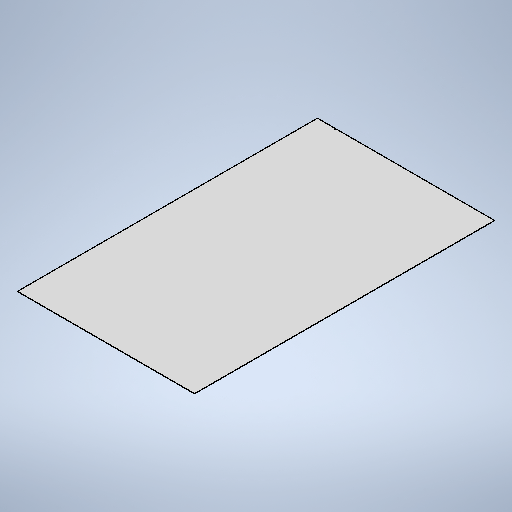
# Autodesk Inventor part: GnG frame 1.1 floor sheet 4
Saved by Autodesk Inventor 2025.3 (Build 293356000, 356)
## iProperties
Created: 2025-10-28
Part Number: GnG frame 1.1 floor sheet 4
Material: Stainless Steel
Document SubType Name: Sheet Metal
Designer: admin
Mass: 280.619 g
Surface Area: 364.406 cm^2
Volume: 35.0774 cm^3
Density: 8 g/cm^3
Sheet Metal Rule: AISI304 3mm Die 32
Sheet Metal Width: 1240,000 mm
Sheet Metal Length: 2100,000 mm
Sheet Metal Area: 2604000,000 mm^2
Appearance: Default
Stock Number: 1.4
Flat Pattern Width: 124 cm
Flat Pattern Length: 210 cm
Flat Pattern Area: 26040 cm^2
Author: admin
Autodesk Inventor part; units mm, degrees
ref_plane "YZ Plane" through (0, 0, 0) normal (1, 0, 0) x (0, 1, 0)
ref_plane "XZ Plane" through (0, 0, 0) normal (0, 1, 0) x (-1, 0, 0)
ref_plane "XY Plane" through (0, 0, 0) normal (0, 0, 1) x (1, 0, 0)
sketch "Sketch1" plane through (0, 0, 0) normal (0, 0, 1) x (1, 0, 0)
  line L0 (0, 0) -> (-1240, 0)
  line L1 (-1240, 0) -> (-1240, -2100)
  line L2 (-1240, -2100) -> (0, -2100)
  line L3 (0, -2100) -> (0, 0)
  line L4 (0, 0) -> (-35, 0)
  line L5 (-35, 0) -> (-35, -35)
  line L6 (-35, -35) -> (0, -35)
  line L7 (0, -35) -> (0, 0)
  line L8 (0, -2100) -> (-35, -2100)
  line L9 (-35, -2100) -> (-35, -2065)
  line L10 (-35, -2065) -> (0, -2065)
  line L11 (0, -2065) -> (0, -2100)
  line L12 (-1240, 0) -> (-1205, 0)
  line L13 (-1205, 0) -> (-1205, -35)
  line L14 (-1205, -35) -> (-1240, -35)
  line L15 (-1240, -35) -> (-1240, 0)
  line L16 (-1240, -2100) -> (-1205, -2100)
  line L17 (-1205, -2100) -> (-1205, -2065)
  line L18 (-1205, -2065) -> (-1240, -2065)
  line L19 (-1240, -2065) -> (-1240, -2100)
  line L20 (-1095, -2100) -> (-1005, -2100)
  line L21 (-1005, -2100) -> (-1005, -2065)
  line L22 (-1005, -2065) -> (-1095, -2065)
  line L23 (-1095, -2065) -> (-1095, -2100)
  line L24 (-1095, 0) -> (-1005, 0)
  line L25 (-1005, 0) -> (-1005, -35)
  line L26 (-1005, -35) -> (-1095, -35)
  line L27 (-1095, -35) -> (-1095, 0)
  point P0 (0, -35)
  point P1 (0, -2065)
  point P2 (-1005, -2100)
  point P3 (-1005, 0)
  dimension "d22" = 1240
  dimension "d23" = 2100
  dimension "d24" = 35
  dimension "d25" = 35
  dimension "d28" = 90
  dimension "d29" = 970
  measures "d22" distance of L2.end L1.end
  measures "d23" distance of L1.end L0.end
  measures "d24" distance of L6.end L5.end
  measures "d25" distance of L5.end L4.end
  measures "d28" distance of L25.end L26.end
  measures "d29" distance between parallel lines of L5 L25
extrude "Plate1" add sketch "Sketch1" along normal blind 3
sketch "Sketch5" plane through (0, 0, 3) normal (0, 0, 1) x (1, 0, 0)
  line L0 (-1135, 0) -> (-1133, 0)
  line L1 (-1131, 0) -> (-1129, 0)
  circle A0 centre (-1140, 0) radius 1.5
  line L2 (-1125, 0) -> (-1125, -5)
  line L3 (-1123, 0) -> (-1121.9884, -4.6072)
  arc A1 (-1121.9884, -4.6072) -> (-1121.0116, -4.6072) centre (-1121.5, -4.5) ccw
  line L4 (-1123, 0) -> (-1120, 0)
  line L5 (-1125, 0) -> (-1123, 0) construction
  line L6 (-1120, 0) -> (-1118, 0) construction
  line L7 (-1121.0116, -4.6072) -> (-1120, 0)
  line L8 (-1118, -5) -> (-1118, 0)
  line L9 (-1118, 0) -> (-1116, 0)
  line L10 (-1116, 0) -> (-1116, -5)
  line L11 (-1116, -5) -> (-1118, -5)
  line L12 (-1116, -2.5) -> (-1114, -2.5) construction
  line L13 (-1129, -5) -> (-1131, -5)
  line L14 (-1125, -5) -> (-1127, -5)
  line L15 (-1129, -2.5) -> (-1127, -2.5) construction
  line L16 (-1133, -2.5) -> (-1131, -2.5) construction
  line L17 (-1127, 0) -> (-1125, 0)
  line L18 (-1127, -5) -> (-1127, 0)
  line L19 (-1129, 0) -> (-1129, -5)
  line L20 (-1131, -5) -> (-1131, 0)
  line L21 (-1133, 0) -> (-1133, -5)
  line L22 (-1135, -5) -> (-1135, 0)
  line L23 (-1133, -5) -> (-1135, -5)
  line L24 (-1114, -5) -> (-1114, 0)
  line L25 (-1112, -5) -> (-1114, -5)
  line L26 (-1114, 0) -> (-1112, 0)
  line L27 (-1112, 0) -> (-1112, -5)
  line L28 (-1112, -2.5) -> (-1110, -2.5) construction
  line L29 (-1110, -5) -> (-1110, 0)
  line L30 (-1110, 0) -> (-1108, 0)
  line L31 (-1108, 0) -> (-1108, -5)
  line L32 (-1108, -5) -> (-1110, -5)
  line L33 (-1240, 0) -> (0, 0) projected
  line L34 (-1104, -5) -> (-1106, -5)
  line L35 (-1106, -5) -> (-1106, 0)
  line L36 (-1104, 0) -> (-1104, -5)
  line L37 (-1106, 0) -> (-1104, 0)
  line L38 (-1106, -2.5) -> (-1108, -2.5)
  point P0 (-1121.5, 0)
  point P1 (-1105, 0)
  point P2 (-1104, 0)
  point P3 (-1106, 0)
  dimension "d30" = 2
  dimension "d31" = 5
  dimension "d32" = 0.5
  dimension "d33" = 3
  dimension "d34" = 2
  dimension "d35" = 5
  dimension "d36" = 3
  dimension "d37" = 5
  dimension "d38" = 100
  constraints: 76 end point, 14 parallel, 13 horizontal, 12 equal length, 12 midpoint, 7 perpendicular, 5 collinear, 3 point on line, 3 tangent, 2 centre point, 2 point on circle, 1 vertical alignment
  measures "d30" distance of L21.end L23.end
  measures "d31" distance of L23.end L0.start
  measures "d32" radius of A1
  measures "d33" distance of L5.end L4.end
  measures "d34" distance of L10.end L8.start
  measures "d35" distance of L8.start L6.end
  measures "d36" diameter of A0
  measures "d37" distance of A0.centre L0.start
  measures "d38" distance of L33.start A0.centre
extrude "Cut1" cut sketch "Sketch5" against normal blind 3 contours L30 L31 L32 L29 | L26 L27 L25 L24 | L9 L10 L11 L8 | A0 L33 | L33 A0 | L33 L36 L34 L35
equation "\"d24\" = d25"
equation "\"d32\" = 0.25 * d30"
equation "\"d39\" = Thickness"
equation "\"d2\" = Thickness"
equation "\"BendReliefWidth\" = Thickness"
equation "\"BendReliefDepth\" = 0.5 * Thickness"
equation "\"CornerReliefSize\" = 4 * Thickness"
equation "\"MinimumRemnant\" = 2 * Thickness"
equation "\"TransitionRadius\" = BendRadius"
equation "\"JacobiRadiusSize\" = BendRadius"
equation "\"GapSize\" = Thickness"
equation "\"Thickness\" = 3"
equation "\"BendRadius\" = 5"
body "Solid1"
